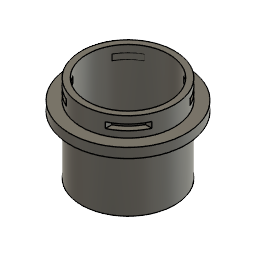
Cold Inlet circular (Autodesk Fusion 360 design; units mm, degrees)
Autodesk Fusion 360 part; units mm, degrees
sketch "Sketch1" plane through (0, 0, 0) normal (0, 0, 1) x (1, 0, 0) in component "sleeve v2 v1"
  circle A0 centre (0, 0) radius 30
  dimension "d1" = 60
  constraint coincident A0.centre origin
  measures "d1" diameter of A0
extrude "Extrude1" add sketch "Sketch1" along normal blind 5 in component "sleeve v2 v1"
sketch "Sketch2" plane through (0, 0, 5) normal (0, 0, 1) x (-1, 0, 0) in component "sleeve v2 v1"
  circle A0 centre (0, 0) radius 30
  circle A1 centre (0, 0) radius 24.1
  dimension "d4" = 48.2
  constraint coincident A0.centre A1.centre
  measures "d4" diameter of A1
extrude "Extrude2" add sketch "Sketch2" along normal blind 25 contours A1 in component "sleeve v2 v1"
sketch "Sketch3" plane through (0, 0, 0) normal (0, 0, -1) x (1, 0, 0) in component "sleeve v2 v1"
  circle A0 centre (0, 0) radius 30
  circle A1 centre (0, 0) radius 24.1
extrude "Extrude3" add sketch "Sketch3" along normal blind 30 contours A1 in component "sleeve v2 v1"
sketch "Sketch4" plane through (0, 0, 30) normal (0, 0, 1) x (-1, 0, 0) in component "sleeve v2 v1"
  circle A0 centre (0, 0) radius 24.1
  circle A1 centre (0, 0) radius 21.1
  dimension "d9" = -3
extrude "Extrude4" cut sketch "Sketch4" against normal blind 60 contours A1 in component "sleeve v2 v1"
extrude "Extrude5" cut 1 faces at (-23.0103, 1.1973, 30) along direction (0, 0, -1) blind 15 in component "sleeve v2 v1"
sketch "Sketch1 (2)" plane through (0, 0, 0) normal (0, 1, 0) x (1, 0, 0)
  line L0 (22.8521, 10.138, 8) -> (18.5049, 10.138, 8)
  line L1 (10, 18.5798, 8) -> (10, 22.9129, 8)
  arc A0 through (22.8521, 10.138, 8) (17.6243, 17.7309, 8) (10, 22.9129, 8)
  arc A1 through (18.5049, 10.138, 8) (14.8643, 14.9754, 8) (10, 18.5798, 8)
  arc A2 through (-10.138, 18.5049, 8) (-14.9754, 14.8643, 8) (-18.5798, 10, 8)
  line L2 (-18.5798, 10, 8) -> (-22.9129, 10, 8)
  arc A3 through (-10.138, 22.8521, 8) (-17.7309, 17.6243, 8) (-22.9129, 10, 8)
  line L3 (-10.138, 22.8521, 8) -> (-10.138, 18.5049, 8)
  arc A4 through (-18.5049, -10.138, 8) (-14.8643, -14.9754, 8) (-10, -18.5798, 8)
  line L4 (-10, -18.5798, 8) -> (-10, -22.9129, 8)
  arc A5 through (-22.8521, -10.138, 8) (-17.6243, -17.7309, 8) (-10, -22.9129, 8)
  line L5 (-22.8521, -10.138, 8) -> (-18.5049, -10.138, 8)
  arc A6 through (10.138, -18.5049, 8) (14.9754, -14.8643, 8) (18.5798, -10, 8)
  line L6 (18.5798, -10, 8) -> (22.9129, -10, 8)
  arc A7 through (10.138, -22.8521, 8) (17.7309, -17.6243, 8) (22.9129, -10, 8)
  line L7 (10.138, -22.8521, 8) -> (10.138, -18.5049, 8)
  dimension "d16" = 42.2
  dimension "d17" = 50
  dimension "d19" = 360
extrude "Extrude6" cut sketch "Sketch1 (2)" along normal blind 3 contours L0 L1 A0 A1 | A2 L2 A3 L3 | A4 L4 A5 L5 | A6 L6 A7 L7 in plane through (0, 8, 0) normal (0, 1, 0) sketch seen with x (1, 0, 0) y (0, 0, 1) z (0, -1, 0) at (0, 0.2727, 0.2727) in component "sleeve v2 v1"
component "sleeve v2 v1" placed x (1, 0, 0) y (0, 0, -1) z (0, 1, 0) at (0, -0.2727, 0.2727)
